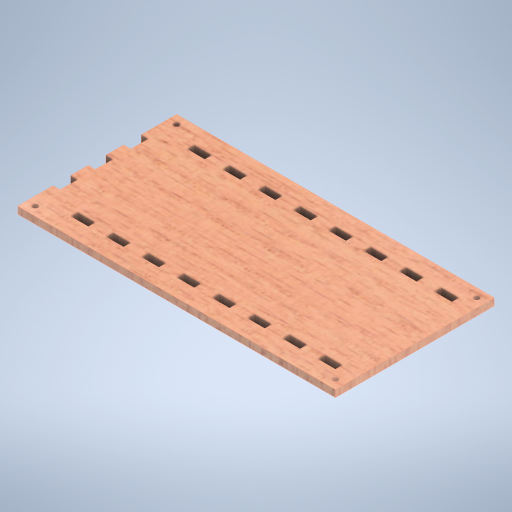
# Autodesk Inventor part: ER_lipo_bottom_1
Saved by Autodesk Inventor 2023 (Build 270158000, 158)
## iProperties
Created: 2023-03-05
Part Number: ER_lipo_bottom_1
Material: 木材 (オーク)
Document SubType Name: Modeling
Designer: mkhr7
Density: 0.76 g/cm^3
Appearance: ホワイト オーク材 - ナチュラル 標準の光沢
Author: mkhr7
Autodesk Inventor part; units mm, degrees
ref_plane "YZ Plane" through (0, 0, 0) normal (1, 0, 0) x (0, 1, 0)
ref_plane "XZ Plane" through (0, 0, 0) normal (0, 1, 0) x (-1, 0, 0)
ref_plane "XY Plane" through (0, 0, 0) normal (0, 0, 1) x (1, 0, 0)
sketch "スケッチ1" plane through (0, 0, 0) normal (0, 1, 0) x (-1, 0, 0)
  line L0 (0, 0) -> (180, 0)
  line L1 (180, 0) -> (180, -90)
  line L2 (180, -90) -> (0, -90)
  line L3 (0, -90) -> (0, 0)
  line L4 (20, -10) -> (10, -10)
  line L5 (10, -10) -> (10, -14)
  line L6 (10, -14) -> (20, -14)
  line L7 (20, -14) -> (20, -10)
  line L8 (20, -76) -> (10, -76)
  line L9 (10, -76) -> (10, -80)
  line L10 (10, -80) -> (20, -80)
  line L11 (20, -80) -> (20, -76)
  line L12 (40, -76) -> (30, -76)
  line L13 (30, -76) -> (30, -80)
  line L14 (30, -80) -> (40, -80)
  line L15 (40, -80) -> (40, -76)
  line L16 (40, -10) -> (30, -10)
  line L17 (30, -10) -> (30, -14)
  line L18 (40, -14) -> (40, -10)
  line L19 (30, -14) -> (40, -14)
  line L20 (60, -76) -> (50, -76)
  line L21 (50, -76) -> (50, -80)
  line L22 (50, -80) -> (60, -80)
  line L23 (60, -80) -> (60, -76)
  line L24 (60, -10) -> (50, -10)
  line L25 (50, -10) -> (50, -14)
  line L26 (60, -14) -> (60, -10)
  line L27 (50, -14) -> (60, -14)
  line L28 (80, -76) -> (70, -76)
  line L29 (70, -76) -> (70, -80)
  line L30 (70, -80) -> (80, -80)
  line L31 (80, -80) -> (80, -76)
  line L32 (80, -10) -> (70, -10)
  line L33 (70, -10) -> (70, -14)
  line L34 (80, -14) -> (80, -10)
  line L35 (70, -14) -> (80, -14)
  line L36 (100, -76) -> (90, -76)
  line L37 (90, -76) -> (90, -80)
  line L38 (90, -80) -> (100, -80)
  line L39 (100, -80) -> (100, -76)
  line L40 (100, -10) -> (90, -10)
  line L41 (90, -10) -> (90, -14)
  line L42 (100, -14) -> (100, -10)
  line L43 (90, -14) -> (100, -14)
  line L44 (120, -76) -> (110, -76)
  line L45 (110, -76) -> (110, -80)
  line L46 (110, -80) -> (120, -80)
  line L47 (120, -80) -> (120, -76)
  line L48 (120, -10) -> (110, -10)
  line L49 (110, -10) -> (110, -14)
  line L50 (120, -14) -> (120, -10)
  line L51 (110, -14) -> (120, -14)
  line L52 (140, -76) -> (130, -76)
  line L53 (130, -76) -> (130, -80)
  line L54 (130, -80) -> (140, -80)
  line L55 (140, -80) -> (140, -76)
  line L56 (140, -10) -> (130, -10)
  line L57 (130, -10) -> (130, -14)
  line L58 (140, -14) -> (140, -10)
  line L59 (130, -14) -> (140, -14)
  line L60 (160, -76) -> (150, -76)
  line L61 (150, -76) -> (150, -80)
  line L62 (150, -80) -> (160, -80)
  line L63 (160, -80) -> (160, -76)
  line L64 (160, -10) -> (150, -10)
  line L65 (150, -10) -> (150, -14)
  line L66 (160, -14) -> (160, -10)
  line L67 (150, -14) -> (160, -14)
  line L68 (180, -20) -> (176, -20)
  line L69 (176, -20) -> (176, -30)
  line L70 (176, -30) -> (180, -30)
  line L71 (180, -30) -> (180, -20)
  line L72 (176, -40) -> (176, -50)
  line L73 (180, -40) -> (176, -40)
  line L74 (176, -50) -> (180, -50)
  line L75 (180, -50) -> (180, -40)
  line L76 (176, -60) -> (176, -70)
  line L77 (180, -60) -> (176, -60)
  line L78 (176, -70) -> (180, -70)
  line L79 (180, -70) -> (180, -60)
  circle A0 centre (5, -5) radius 1.55
  circle A1 centre (5, -85) radius 1.55
  circle A2 centre (175, -85) radius 1.55
  circle A3 centre (175, -5) radius 1.55
  point P0 (10, -78)
  point P1 (30, -78)
  point P2 (50, -78)
  point P3 (70, -78)
  point P4 (90, -78)
  point P5 (110, -78)
  point P6 (130, -78)
  point P7 (150, -78)
  dimension "d0" = 180
  dimension "d1" = 90
  dimension "d2" = 10
  dimension "d3" = 4
  dimension "d4" = 10
  dimension "d5" = 10
  dimension "d6" = 10
  dimension "d7" = 4
  dimension "d8" = 10
  dimension "d9" = 10
  dimension "d12" = 20
  dimension "d17" = 4
  dimension "d18" = 10
  dimension "d19" = 20
  dimension "d22" = 20
  dimension "d27" = 0
  dimension "d28" = 3.1
  dimension "d29" = 3.1
  dimension "d30" = 3.1
  dimension "d31" = 3.1
  dimension "d32" = 5
  dimension "d33" = 5
  dimension "d34" = 5
  dimension "d35" = 5
  dimension "d36" = 5
  dimension "d37" = 5
  dimension "d39" = 5
  dimension "d40" = 5
  constraints: 160 end point, 8 parallel, 5 horizontal, 4 centre point, 4 perpendicular, 1 midpoint, 1 vertical, 135 other
  measures "d0" distance of L1.end L2.end
  measures "d1" distance of L0.end L1.end
  measures "d2" distance of L6.end L5.end
  measures "d3" distance of L5.end L4.end
  measures "d4" distance between parallel lines of L0 L4
  measures "d5" distance between parallel lines of L3 L5
  measures "d6" distance of L10.end L9.end
  measures "d7" distance of L9.end L8.end
  measures "d8" distance between parallel lines of L2 L10
  measures "d9" distance from line of point (10, -78) L3
  measures "d12" distance of L8.start L12.start
  measures "d17" distance of L70.end L69.end
  measures "d18" distance of L69.end L68.end
  measures "d19" distance between parallel lines of L0 L68
  measures "d22" distance of L68.end L72.start
  measures "d27" distance between parallel lines of L1 L71
  measures "d28" diameter of A0
  measures "d29" diameter of A1
  measures "d30" diameter of A2
  measures "d31" diameter of A3
  measures "d32" distance from line of L1 A3.centre
  measures "d33" distance from line of L0 A3.centre
  measures "d34" distance from line of L2 A2.centre
  measures "d35" distance from line of L1 A2.centre
  measures "d36" distance from line of L3 A1.centre
  measures "d37" distance from line of L2 A1.centre
  measures "d39" distance from line of L0 A0.centre
  measures "d40" distance from line of L3 A0.centre
extrude "押し出し1" add sketch "スケッチ1" along normal blind 4 contours L0 L1 L68 L69 L70 L73 L72 L74 L77 L76 L78 L2 L3
